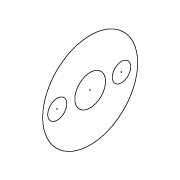
# Autodesk Inventor part: MotorSpacer
Saved by Autodesk Inventor 2013 SP1 (Build 170176100, 176)
## iProperties
Created: 2013-12-03
Part Number: MotorSpacer
Material: ABS Plastic
Document SubType Name: Sheet Metal
Designer: robotics
Density: 1.06 g/cm^3
Sheet Metal Rule: Acrylic 3mm
Author: robotics
Autodesk Inventor part; units mm, degrees
ref_plane "YZ Plane" through (0, 0, 0) normal (1, 0, 0) x (0, 1, 0)
ref_plane "XZ Plane" through (0, 0, 0) normal (0, 1, 0) x (-1, 0, 0)
ref_plane "XY Plane" through (0, 0, 0) normal (0, 0, 1) x (1, 0, 0)
sketch "Sketch1" plane through (0, 0, 0) normal (1, 0, 0) x (0, 1, 0)
  circle A0 centre (0, 0) radius 30.48
  circle A1 centre (0, 0) radius 9.525
  circle A2 centre (25.3286, -1.9038) radius 3
  circle A3 centre (-25.3286, 1.9038) radius 3
  circle A4 centre (0, -33.0962) radius 11.43
  line L0 (27.3765, 13.4) -> (-27.3765, 13.4)
  line L1 (-25.3286, 1.9038) -> (25.3286, -1.9038) construction
  line L2 (0, -33.0962) -> (-25.3286, -33.0962)
  point P0 (10.5127, -28.6097)
  point P1 (-10.5127, -28.6097)
  dimension "d0" = 6
  dimension "d2" = 19.05
  dimension "d3" = 60.96
  dimension "d6" = 22.86
  dimension "d8" = 50.8
  dimension "d9" = 13.4
  dimension "d11" = 70
  dimension "d12" = 33.0962
  measures "d0" diameter of A3
  measures "d2" diameter of A1
  measures "d3" diameter of A0
  measures "d6" diameter of A4
  measures "d8" distance of L1.start L1.end
  measures "d9" distance from line of point (0, 0) L0
  measures "d11" diameter of L1.start L2
  measures "d12" distance of point (0, 0) L2.start
extrude "Plate1" add sketch "Sketch1" along normal blind 3 contours A0 A4 L0
equation "\"BendRadius\" = Thickness"
equation "\"BendReliefWidth\" = Thickness"
equation "\"BendReliefDepth\" = 0.5 * Thickness"
equation "\"CornerReliefSize\" = 4 * Thickness"
equation "\"MinimumRemnant\" = 2 * Thickness"
equation "\"TransitionRadius\" = BendRadius"
equation "\"JacobiRadiusSize\" = BendRadius"
equation "\"GapSize\" = Thickness"
equation "\"d7\" = BendRadius"
equation "\"Thickness\" = 3"
body "Solid1"
